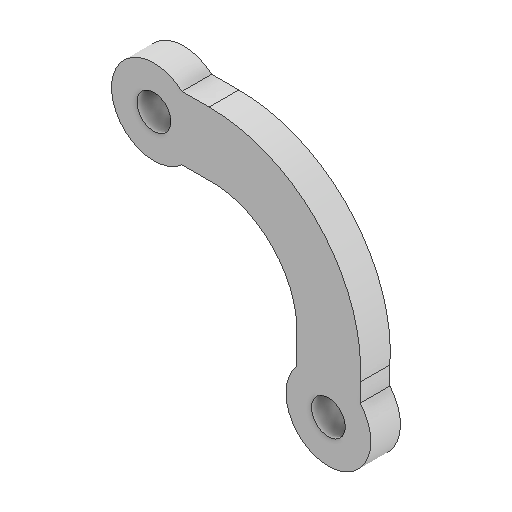
# Autodesk Inventor part: Push Arm
Saved by Autodesk Inventor 2025 (Build 290162010, 162A)
## iProperties
Created: 2024-12-05
Part Number: Push Arm
Material: Generic
Document SubType Name: Modeling
Designer: ALEXANDERNICHOLS
Density: 1 g/cm^3
Appearance: Default
Author: ALEXANDERNICHOLS
Autodesk Inventor part; units mm, degrees
ref_plane "YZ Plane" through (0, 0, 0) normal (1, 0, 0) x (0, 1, 0)
ref_plane "XZ Plane" through (0, 0, 0) normal (0, 1, 0) x (-1, 0, 0)
ref_plane "XY Plane" through (0, 0, 0) normal (0, 0, 1) x (1, 0, 0)
sketch "Sketch1" plane through (0, 0, 0) normal (0, 0, 1) x (1, 0, 0)
  circle A0 centre (0, 0) radius 2.032
  circle A1 centre (0, 0) radius 5.08
  line L0 (3.81, 3.3601) -> (3.81, 5.5534)
  line L1 (-3.81, 3.3601) -> (-3.81, 6.2503)
  circle A2 centre (-20.9, 21.2222) radius 2.032
  circle A3 centre (-20.9, 21.2222) radius 5.08
  line L2 (-17.5399, 25.0322) -> (-14.2921, 25.0322)
  line L3 (-17.5399, 17.4122) -> (-14.7055, 17.4122)
  arc A4 (-3.81, 6.2503) -> (-14.7055, 17.4122) centre (-14.0813, 7.1228) ccw
  arc A5 (3.81, 5.5534) -> (-14.2921, 25.0322) centre (-14.2921, 6.8814) ccw
  point P0 (-3.81, 4.8052)
  dimension "d0" = 4.064
  dimension "d1" = 10.16
  dimension "d2" = 7.62
  dimension "d3" = 3.81
  dimension "d4" = 4.064
  dimension "d5" = 10.16
  dimension "d6" = 7.62
  dimension "d7" = 3.81
  constraints: 8 end point, 8 point on circle, 6 centre point, 3 coincident, 2 horizontal, 2 vertical, 1 midpoint, 1 tangent
  measures "d0" diameter of A0
  measures "d1" diameter of A1
  measures "d2" distance from line of L0 point (-3.81, 4.805)
  measures "d3" distance from line of point (0, 0) L0
  measures "d4" diameter of A2
  measures "d5" diameter of A3
  measures "d6" distance between parallel lines of L3 L2
  measures "d7" distance from line of A2.centre L3
extrude "Extrusion1" add sketch "Sketch1" along normal blind 3.556
equation "\"d3\" = 0.5 * d2"
equation "\"d7\" = 0.5 * d6"
body "Solid1"
